mid (Autodesk Fusion 360 design; units mm, degrees)
Autodesk Fusion 360 part; units mm, degrees
note: some values were not read from the file. Set by a fixed rule: which sketch regions a step uses.
sketch "Sketch1" plane through (0, 0, 0) normal (0, 1, 0) x (1, 0, 0)
  line L0 (0, 0) -> (-60, 0)
  line L1 (-60, 0) -> (-60, -40)
  line L2 (-60, -40) -> (0, -40)
  line L3 (0, -40) -> (0, 0)
  spline S0 degree 2 poles (-31.401, -19.5282) (-31.401, -20.0578) (-31.6754, -20.3466) knots 0 0 0 1 1 1
  spline S1 degree 2 poles (-31.6754, -20.3466) (-31.9498, -20.6355) (-32.4457, -20.6355) knots 0 0 0 1 1 1
  spline S2 degree 2 poles (-32.4457, -20.6355) (-32.903, -20.6355) (-33.1534, -20.3563) knots 0 0 0 1 1 1
  spline S3 degree 2 poles (-33.1534, -20.3563) (-33.4037, -20.077) (-33.4037, -19.5667) knots 0 0 0 1 1 1
  line L4 (-33.4037, -19.5667) -> (-33.6011, -20.5296)
  spline S4 degree 2 poles (-33.6011, -20.5296) (-33.3652, -21.0254) (-32.9776, -21.2975) knots 0 0 0 1 1 1
  spline S5 degree 2 poles (-32.9776, -21.2975) (-32.5901, -21.5695) (-32.1231, -21.5695) knots 0 0 0 1 1 1
  spline S6 degree 2 poles (-32.1231, -21.5695) (-31.5839, -21.5695) (-31.2012, -21.3312) knots 0 0 0 1 1 1
  spline S7 degree 2 poles (-31.2012, -21.3312) (-30.8184, -21.0928) (-30.6186, -20.6355) knots 0 0 0 1 1 1
  spline S8 degree 2 poles (-30.6186, -20.6355) (-30.4188, -20.1781) (-30.4188, -19.533) knots 0 0 0 1 1 1
  line L5 (-30.4188, -19.533) -> (-30.4188, -16.5)
  line L6 (-30.4188, -16.5) -> (-31.401, -16.5)
  line L7 (-31.401, -16.5) -> (-31.401, -19.5282)
  line L8 (-37.3707, -21.4972) -> (-36.3886, -21.4972)
  line L9 (-36.3886, -21.4972) -> (-36.3886, -16.5)
  line L10 (-36.3886, -16.5) -> (-37.3707, -16.5)
  line L11 (-37.3707, -16.5) -> (-37.3707, -21.4972)
  spline S9 degree 2 poles (-34.3858, -19.5282) (-34.3858, -20.0578) (-34.6458, -20.3466) knots 0 0 0 1 1 1
  spline S10 degree 2 poles (-34.6458, -20.3466) (-34.9058, -20.6355) (-35.3824, -20.6355) knots 0 0 0 1 1 1
  spline S11 degree 2 poles (-35.3824, -20.6355) (-35.8638, -20.6355) (-36.1262, -20.3803) knots 0 0 0 1 1 1
  spline S12 degree 2 poles (-36.1262, -20.3803) (-36.3886, -20.1252) (-36.3886, -19.663) knots 0 0 0 1 1 1
  line L12 (-36.3886, -19.663) -> (-36.4897, -20.6259)
  spline S13 degree 2 poles (-36.4897, -20.6259) (-36.2586, -21.0784) (-35.8855, -21.3239) knots 0 0 0 1 1 1
  spline S14 degree 2 poles (-35.8855, -21.3239) (-35.5124, -21.5695) (-35.0598, -21.5695) knots 0 0 0 1 1 1
  spline S15 degree 2 poles (-35.0598, -21.5695) (-34.5351, -21.5695) (-34.1644, -21.3312) knots 0 0 0 1 1 1
  spline S16 degree 2 poles (-34.1644, -21.3312) (-33.7937, -21.0928) (-33.5987, -20.6355) knots 0 0 0 1 1 1
  spline S17 degree 2 poles (-33.5987, -20.6355) (-33.4037, -20.1781) (-33.4037, -19.533) knots 0 0 0 1 1 1
  line L13 (-33.4037, -19.533) -> (-33.4037, -16.5)
  line L14 (-33.4037, -16.5) -> (-34.3858, -16.5)
  line L15 (-34.3858, -16.5) -> (-34.3858, -19.5282)
  line L16 (-28.9264, -23.5) -> (-27.9443, -23.5)
  line L17 (-27.9443, -23.5) -> (-27.9443, -22.5179)
  line L18 (-27.9443, -22.5179) -> (-28.9264, -22.5179)
  line L19 (-28.9264, -22.5179) -> (-28.9264, -23.5)
  line L20 (-28.9264, -21.4972) -> (-27.9443, -21.4972)
  line L21 (-27.9443, -21.4972) -> (-27.9443, -16.5)
  line L22 (-27.9443, -16.5) -> (-28.9264, -16.5)
  line L23 (-28.9264, -16.5) -> (-28.9264, -21.4972)
  line L24 (-23.6114, -23.5) -> (-22.6293, -23.5)
  line L25 (-22.6293, -23.5) -> (-22.6293, -16.5)
  line L26 (-22.6293, -16.5) -> (-23.6114, -16.5)
  line L27 (-23.6114, -16.5) -> (-23.6114, -23.5)
  spline S18 degree 2 poles (-24.868, -16.4133) (-25.4168, -16.4133) (-25.8043, -16.6516) knots 0 0 0 1 1 1
  spline S19 degree 2 poles (-25.8043, -16.6516) (-26.1919, -16.89) (-26.3941, -17.3473) knots 0 0 0 1 1 1
  spline S20 degree 2 poles (-26.3941, -17.3473) (-26.5963, -17.8047) (-26.5963, -18.445) knots 0 0 0 1 1 1
  line L28 (-26.5963, -18.445) -> (-26.5963, -19.5475)
  spline S21 degree 2 poles (-26.5963, -19.5475) (-26.5963, -20.1926) (-26.3989, -20.6499) knots 0 0 0 1 1 1
  spline S22 degree 2 poles (-26.3989, -20.6499) (-26.2015, -21.1073) (-25.8236, -21.3456) knots 0 0 0 1 1 1
  spline S23 degree 2 poles (-25.8236, -21.3456) (-25.4457, -21.5839) (-24.9161, -21.5839) knots 0 0 0 1 1 1
  spline S24 degree 2 poles (-24.9161, -21.5839) (-24.4732, -21.5839) (-24.1049, -21.3528) knots 0 0 0 1 1 1
  spline S25 degree 2 poles (-24.1049, -21.3528) (-23.7366, -21.1217) (-23.5103, -20.7029) knots 0 0 0 1 1 1
  line L29 (-23.5103, -20.7029) -> (-23.6114, -19.6823)
  spline S26 degree 2 poles (-23.6114, -19.6823) (-23.6114, -20) (-23.727, -20.2263) knots 0 0 0 1 1 1
  spline S27 degree 2 poles (-23.727, -20.2263) (-23.8425, -20.4525) (-24.0616, -20.5705) knots 0 0 0 1 1 1
  spline S28 degree 2 poles (-24.0616, -20.5705) (-24.2806, -20.6884) (-24.5935, -20.6884) knots 0 0 0 1 1 1
  spline S29 degree 2 poles (-24.5935, -20.6884) (-25.0798, -20.6884) (-25.347, -20.3851) knots 0 0 0 1 1 1
  spline S30 degree 2 poles (-25.347, -20.3851) (-25.6142, -20.0818) (-25.6142, -19.533) knots 0 0 0 1 1 1
  line L30 (-25.6142, -19.533) -> (-25.6142, -18.445)
  spline S31 degree 2 poles (-25.6142, -18.445) (-25.6142, -17.901) (-25.347, -17.6049) knots 0 0 0 1 1 1
  spline S32 degree 2 poles (-25.347, -17.6049) (-25.0798, -17.3088) (-24.5935, -17.3088) knots 0 0 0 1 1 1
  spline S33 degree 2 poles (-24.5935, -17.3088) (-24.2806, -17.3088) (-24.0616, -17.4316) knots 0 0 0 1 1 1
  spline S34 degree 2 poles (-24.0616, -17.4316) (-23.8425, -17.5543) (-23.727, -17.7854) knots 0 0 0 1 1 1
  spline S35 degree 2 poles (-23.727, -17.7854) (-23.6114, -18.0165) (-23.6114, -18.3391) knots 0 0 0 1 1 1
  line L31 (-23.6114, -18.3391) -> (-23.544, -17.2847)
  spline S36 degree 2 poles (-23.544, -17.2847) (-23.6933, -16.914) (-24.0327, -16.6637) knots 0 0 0 1 1 1
  spline S37 degree 2 poles (-24.0327, -16.6637) (-24.3721, -16.4133) (-24.868, -16.4133) knots 0 0 0 1 1 1
  line L32 (0, 5) -> (-60, 5)
  line L33 (-60, 5) -> (-60, 33)
  line L34 (-60, 33) -> (0, 33)
  line L35 (0, 33) -> (0, 5)
  spline S38 degree 2 poles (-47.8102, 16.7607) (-48.641, 16.7607) (-49.271, 16.392) knots 0 0 0 1 1 1
  spline S39 degree 2 poles (-49.271, 16.392) (-49.901, 16.0234) (-50.2476, 15.3466) knots 0 0 0 1 1 1
  spline S40 degree 2 poles (-50.2476, 15.3466) (-50.5942, 14.6699) (-50.5942, 13.7785) knots 0 0 0 1 1 1
  line L36 (-50.5942, 13.7785) -> (-50.5942, 11.5832)
  spline S41 degree 2 poles (-50.5942, 11.5832) (-50.5942, 10.6919) (-50.2476, 10.0151) knots 0 0 0 1 1 1
  spline S42 degree 2 poles (-50.2476, 10.0151) (-49.901, 9.3384) (-49.271, 8.967) knots 0 0 0 1 1 1
  spline S43 degree 2 poles (-49.271, 8.967) (-48.641, 8.5956) (-47.8102, 8.5956) knots 0 0 0 1 1 1
  spline S44 degree 2 poles (-47.8102, 8.5956) (-47.1224, 8.5956) (-46.5447, 8.89) knots 0 0 0 1 1 1
  spline S45 degree 2 poles (-46.5447, 8.89) (-45.967, 9.1843) (-45.5791, 9.7235) knots 0 0 0 1 1 1
  spline S46 degree 2 poles (-45.5791, 9.7235) (-45.1912, 10.2627) (-45.0536, 10.9725) knots 0 0 0 1 1 1
  line L37 (-45.0536, 10.9725) -> (-46.2036, 10.9725)
  spline S47 degree 2 poles (-46.2036, 10.9725) (-46.3081, 10.5983) (-46.553, 10.304) knots 0 0 0 1 1 1
  spline S48 degree 2 poles (-46.553, 10.304) (-46.7978, 10.0096) (-47.1279, 9.8501) knots 0 0 0 1 1 1
  spline S49 degree 2 poles (-47.1279, 9.8501) (-47.458, 9.6905) (-47.8102, 9.6905) knots 0 0 0 1 1 1
  spline S50 degree 2 poles (-47.8102, 9.6905) (-48.2999, 9.6905) (-48.6685, 9.9271) knots 0 0 0 1 1 1
  spline S51 degree 2 poles (-48.6685, 9.9271) (-49.0371, 10.1637) (-49.2407, 10.5901) knots 0 0 0 1 1 1
  spline S52 degree 2 poles (-49.2407, 10.5901) (-49.4443, 11.0165) (-49.4443, 11.5832) knots 0 0 0 1 1 1
  line L38 (-49.4443, 11.5832) -> (-49.4443, 13.7785)
  spline S53 degree 2 poles (-49.4443, 13.7785) (-49.4443, 14.3398) (-49.2407, 14.7689) knots 0 0 0 1 1 1
  spline S54 degree 2 poles (-49.2407, 14.7689) (-49.0371, 15.1981) (-48.6685, 15.4319) knots 0 0 0 1 1 1
  spline S55 degree 2 poles (-48.6685, 15.4319) (-48.2999, 15.6657) (-47.8102, 15.6657) knots 0 0 0 1 1 1
  spline S56 degree 2 poles (-47.8102, 15.6657) (-47.4525, 15.6657) (-47.1252, 15.5172) knots 0 0 0 1 1 1
  spline S57 degree 2 poles (-47.1252, 15.5172) (-46.7978, 15.3686) (-46.553, 15.077) knots 0 0 0 1 1 1
  spline S58 degree 2 poles (-46.553, 15.077) (-46.3081, 14.7854) (-46.2036, 14.3838) knots 0 0 0 1 1 1
  line L39 (-46.2036, 14.3838) -> (-45.0536, 14.3838)
  spline S59 degree 2 poles (-45.0536, 14.3838) (-45.1912, 15.0935) (-45.5818, 15.6327) knots 0 0 0 1 1 1
  spline S60 degree 2 poles (-45.5818, 15.6327) (-45.9725, 16.1719) (-46.5502, 16.4663) knots 0 0 0 1 1 1
  spline S61 degree 2 poles (-46.5502, 16.4663) (-47.1279, 16.7607) (-47.8102, 16.7607) knots 0 0 0 1 1 1
  spline S62 degree 2 poles (-41.2297, 16.7607) (-42.022, 16.7607) (-42.5832, 16.4635) knots 0 0 0 1 1 1
  spline S63 degree 2 poles (-42.5832, 16.4635) (-43.1444, 16.1664) (-43.4388, 15.5915) knots 0 0 0 1 1 1
  spline S64 degree 2 poles (-43.4388, 15.5915) (-43.7332, 15.0165) (-43.7332, 14.2022) knots 0 0 0 1 1 1
  line L40 (-43.7332, 14.2022) -> (-43.7332, 13.5585)
  spline S65 degree 2 poles (-43.7332, 13.5585) (-43.7332, 12.7111) (-43.4498, 12.1114) knots 0 0 0 1 1 1
  spline S66 degree 2 poles (-43.4498, 12.1114) (-43.1664, 11.5117) (-42.6272, 11.1981) knots 0 0 0 1 1 1
  spline S67 degree 2 poles (-42.6272, 11.1981) (-42.088, 10.8845) (-41.3287, 10.8845) knots 0 0 0 1 1 1
  spline S68 degree 2 poles (-41.3287, 10.8845) (-40.6135, 10.8845) (-40.1073, 11.2421) knots 0 0 0 1 1 1
  spline S69 degree 2 poles (-40.1073, 11.2421) (-39.6011, 11.5997) (-39.3343, 12.2765) knots 0 0 0 1 1 1
  spline S70 degree 2 poles (-39.3343, 12.2765) (-39.0674, 12.9532) (-39.0674, 13.8996) knots 0 0 0 1 1 1
  line L41 (-39.0674, 13.8996) -> (-39.0674, 14.2737)
  line L42 (-39.0674, 14.2737) -> (-42.9188, 14.2737)
  line L43 (-42.9188, 14.2737) -> (-42.9188, 13.3714)
  line L44 (-42.9188, 13.3714) -> (-40.1348, 13.3714)
  spline S71 degree 2 poles (-40.1348, 13.3714) (-40.1843, 12.6726) (-40.4952, 12.2847) knots 0 0 0 1 1 1
  spline S72 degree 2 poles (-40.4952, 12.2847) (-40.8061, 11.8968) (-41.3287, 11.8968) knots 0 0 0 1 1 1
  spline S73 degree 2 poles (-41.3287, 11.8968) (-41.967, 11.8968) (-42.3164, 12.315) knots 0 0 0 1 1 1
  spline S74 degree 2 poles (-42.3164, 12.315) (-42.6658, 12.7332) (-42.6658, 13.4979) knots 0 0 0 1 1 1
  line L45 (-42.6658, 13.4979) -> (-42.6658, 14.2242)
  spline S75 degree 2 poles (-42.6658, 14.2242) (-42.6658, 14.934) (-42.2916, 15.3136) knots 0 0 0 1 1 1
  spline S76 degree 2 poles (-42.2916, 15.3136) (-41.9175, 15.6933) (-41.2297, 15.6933) knots 0 0 0 1 1 1
  spline S77 degree 2 poles (-41.2297, 15.6933) (-40.8886, 15.6933) (-40.553, 15.5557) knots 0 0 0 1 1 1
  spline S78 degree 2 poles (-40.553, 15.5557) (-40.2173, 15.4182) (-39.9532, 15.1706) knots 0 0 0 1 1 1
  line L46 (-39.9532, 15.1706) -> (-39.216, 15.9078)
  spline S79 degree 2 poles (-39.216, 15.9078) (-39.6396, 16.315) (-40.1678, 16.5378) knots 0 0 0 1 1 1
  spline S80 degree 2 poles (-40.1678, 16.5378) (-40.696, 16.7607) (-41.2297, 16.7607) knots 0 0 0 1 1 1
  line L47 (-37.5268, 10.967) -> (-36.4044, 10.967)
  line L48 (-36.4044, 10.967) -> (-36.4044, 16.6781)
  line L49 (-36.4044, 16.6781) -> (-37.5268, 16.6781)
  line L50 (-37.5268, 16.6781) -> (-37.5268, 10.967)
  spline S81 degree 2 poles (-34.3851, 12.3205) (-34.5337, 12.1389) (-34.7593, 12.0454) knots 0 0 0 1 1 1
  spline S82 degree 2 poles (-34.7593, 12.0454) (-34.9849, 11.9519) (-35.282, 11.9519) knots 0 0 0 1 1 1
  spline S83 degree 2 poles (-35.282, 11.9519) (-35.8157, 11.9519) (-36.11, 12.2462) knots 0 0 0 1 1 1
  spline S84 degree 2 poles (-36.11, 12.2462) (-36.4044, 12.5406) (-36.4044, 13.0633) knots 0 0 0 1 1 1
  line L51 (-36.4044, 13.0633) -> (-36.5199, 11.9629)
  spline S85 degree 2 poles (-36.5199, 11.9629) (-36.2558, 11.4512) (-35.8377, 11.1678) knots 0 0 0 1 1 1
  spline S86 degree 2 poles (-35.8377, 11.1678) (-35.4195, 10.8845) (-34.9133, 10.8845) knots 0 0 0 1 1 1
  spline S87 degree 2 poles (-34.9133, 10.8845) (-34.5227, 10.8845) (-34.2063, 10.9972) knots 0 0 0 1 1 1
  spline S88 degree 2 poles (-34.2063, 10.9972) (-33.89, 11.11) (-33.6534, 11.3301) knots 0 0 0 1 1 1
  line L52 (-33.6534, 11.3301) -> (-34.3851, 12.3205)
  spline S89 degree 2 poles (-31.2325, 16.7056) (-31.9257, 16.7056) (-32.2476, 16.3232) knots 0 0 0 1 1 1
  spline S90 degree 2 poles (-32.2476, 16.3232) (-32.5695, 15.9409) (-32.5695, 15.1926) knots 0 0 0 1 1 1
  line L53 (-32.5695, 15.1926) -> (-32.5695, 9.3054)
  line L54 (-32.5695, 9.3054) -> (-31.447, 9.3054)
  line L55 (-31.447, 9.3054) -> (-31.447, 15.2036)
  spline S91 degree 2 poles (-31.447, 15.2036) (-31.447, 15.4127) (-31.3645, 15.5254) knots 0 0 0 1 1 1
  spline S92 degree 2 poles (-31.3645, 15.5254) (-31.282, 15.6382) (-31.1224, 15.6382) knots 0 0 0 1 1 1
  line L56 (-31.1224, 15.6382) -> (-30.5832, 15.6382)
  line L57 (-30.5832, 15.6382) -> (-30.5832, 16.7056)
  line L58 (-30.5832, 16.7056) -> (-31.2325, 16.7056)
  line L59 (-33.1582, 10.967) -> (-30.5832, 10.967)
  line L60 (-30.5832, 10.967) -> (-30.5832, 11.9794)
  line L61 (-30.5832, 11.9794) -> (-33.1582, 11.9794)
  line L62 (-33.1582, 11.9794) -> (-33.1582, 10.967)
  line L63 (-29.0426, 8.6781) -> (-27.9202, 8.6781)
  line L64 (-27.9202, 8.6781) -> (-27.9202, 9.8006)
  line L65 (-27.9202, 9.8006) -> (-29.0426, 9.8006)
  line L66 (-29.0426, 9.8006) -> (-29.0426, 8.6781)
  line L67 (-29.0426, 10.967) -> (-27.9202, 10.967)
  line L68 (-27.9202, 10.967) -> (-27.9202, 16.6781)
  line L69 (-27.9202, 16.6781) -> (-29.0426, 16.6781)
  line L70 (-29.0426, 16.6781) -> (-29.0426, 10.967)
  spline S93 degree 2 poles (-26.0495, 10.1912) (-26.0495, 9.4319) (-25.7001, 9.055) knots 0 0 0 1 1 1
  spline S94 degree 2 poles (-25.7001, 9.055) (-25.3508, 8.6781) (-24.6245, 8.6781) knots 0 0 0 1 1 1
  line L71 (-24.6245, 8.6781) -> (-23.7992, 8.6781)
  line L72 (-23.7992, 8.6781) -> (-23.7992, 9.7455)
  line L73 (-23.7992, 9.7455) -> (-24.6025, 9.7455)
  spline S95 degree 2 poles (-24.6025, 9.7455) (-24.762, 9.7455) (-24.8446, 9.8666) knots 0 0 0 1 1 1
  spline S96 degree 2 poles (-24.8446, 9.8666) (-24.9271, 9.9876) (-24.9271, 10.1802) knots 0 0 0 1 1 1
  line L74 (-24.9271, 10.1802) -> (-24.9271, 16.6781)
  line L75 (-24.9271, 16.6781) -> (-26.0495, 16.6781)
  line L76 (-26.0495, 16.6781) -> (-26.0495, 10.1912)
  line L77 (-26.6547, 10.967) -> (-23.7992, 10.967)
  line L78 (-23.7992, 10.967) -> (-23.7992, 11.9243)
  line L79 (-23.7992, 11.9243) -> (-26.6547, 11.9243)
  line L80 (-26.6547, 11.9243) -> (-26.6547, 10.967)
  line L81 (-22.6437, 8.6781) -> (-21.5213, 8.6781)
  line L82 (-21.5213, 8.6781) -> (-21.5213, 9.8006)
  line L83 (-21.5213, 9.8006) -> (-22.6437, 9.8006)
  line L84 (-22.6437, 9.8006) -> (-22.6437, 8.6781)
  line L85 (-22.6437, 10.967) -> (-21.5213, 10.967)
  line L86 (-21.5213, 10.967) -> (-21.5213, 16.6781)
  line L87 (-21.5213, 16.6781) -> (-22.6437, 16.6781)
  line L88 (-22.6437, 16.6781) -> (-22.6437, 10.967)
  spline S97 degree 2 poles (-17.4773, 16.7607) (-18.2696, 16.7607) (-18.8308, 16.4635) knots 0 0 0 1 1 1
  spline S98 degree 2 poles (-18.8308, 16.4635) (-19.392, 16.1664) (-19.6864, 15.5915) knots 0 0 0 1 1 1
  spline S99 degree 2 poles (-19.6864, 15.5915) (-19.9807, 15.0165) (-19.9807, 14.2022) knots 0 0 0 1 1 1
  line L89 (-19.9807, 14.2022) -> (-19.9807, 13.5585)
  spline S100 degree 2 poles (-19.9807, 13.5585) (-19.9807, 12.7111) (-19.6974, 12.1114) knots 0 0 0 1 1 1
  spline S101 degree 2 poles (-19.6974, 12.1114) (-19.414, 11.5117) (-18.8748, 11.1981) knots 0 0 0 1 1 1
  spline S102 degree 2 poles (-18.8748, 11.1981) (-18.3356, 10.8845) (-17.5763, 10.8845) knots 0 0 0 1 1 1
  spline S103 degree 2 poles (-17.5763, 10.8845) (-16.8611, 10.8845) (-16.3549, 11.2421) knots 0 0 0 1 1 1
  spline S104 degree 2 poles (-16.3549, 11.2421) (-15.8487, 11.5997) (-15.5818, 12.2765) knots 0 0 0 1 1 1
  spline S105 degree 2 poles (-15.5818, 12.2765) (-15.315, 12.9532) (-15.315, 13.8996) knots 0 0 0 1 1 1
  line L90 (-15.315, 13.8996) -> (-15.315, 14.2737)
  line L91 (-15.315, 14.2737) -> (-19.1664, 14.2737)
  line L92 (-19.1664, 14.2737) -> (-19.1664, 13.3714)
  line L93 (-19.1664, 13.3714) -> (-16.3824, 13.3714)
  spline S106 degree 2 poles (-16.3824, 13.3714) (-16.4319, 12.6726) (-16.7428, 12.2847) knots 0 0 0 1 1 1
  spline S107 degree 2 poles (-16.7428, 12.2847) (-17.0536, 11.8968) (-17.5763, 11.8968) knots 0 0 0 1 1 1
  spline S108 degree 2 poles (-17.5763, 11.8968) (-18.2146, 11.8968) (-18.564, 12.315) knots 0 0 0 1 1 1
  spline S109 degree 2 poles (-18.564, 12.315) (-18.9133, 12.7332) (-18.9133, 13.4979) knots 0 0 0 1 1 1
  line L94 (-18.9133, 13.4979) -> (-18.9133, 14.2242)
  spline S110 degree 2 poles (-18.9133, 14.2242) (-18.9133, 14.934) (-18.5392, 15.3136) knots 0 0 0 1 1 1
  spline S111 degree 2 poles (-18.5392, 15.3136) (-18.1651, 15.6933) (-17.4773, 15.6933) knots 0 0 0 1 1 1
  spline S112 degree 2 poles (-17.4773, 15.6933) (-17.1362, 15.6933) (-16.8005, 15.5557) knots 0 0 0 1 1 1
  spline S113 degree 2 poles (-16.8005, 15.5557) (-16.4649, 15.4182) (-16.2008, 15.1706) knots 0 0 0 1 1 1
  line L95 (-16.2008, 15.1706) -> (-15.4636, 15.9078)
  spline S114 degree 2 poles (-15.4636, 15.9078) (-15.8872, 16.315) (-16.4154, 16.5378) knots 0 0 0 1 1 1
  spline S115 degree 2 poles (-16.4154, 16.5378) (-16.9436, 16.7607) (-17.4773, 16.7607) knots 0 0 0 1 1 1
  line L96 (-10.5282, 8.6781) -> (-9.4058, 8.6781)
  line L97 (-9.4058, 8.6781) -> (-9.4058, 16.6781)
  line L98 (-9.4058, 16.6781) -> (-10.5282, 16.6781)
  line L99 (-10.5282, 16.6781) -> (-10.5282, 8.6781)
  spline S116 degree 2 poles (-11.9642, 16.7772) (-12.5915, 16.7772) (-13.0344, 16.5048) knots 0 0 0 1 1 1
  spline S117 degree 2 poles (-13.0344, 16.5048) (-13.4773, 16.2325) (-13.7084, 15.7098) knots 0 0 0 1 1 1
  spline S118 degree 2 poles (-13.7084, 15.7098) (-13.9395, 15.1871) (-13.9395, 14.4553) knots 0 0 0 1 1 1
  line L100 (-13.9395, 14.4553) -> (-13.9395, 13.1953)
  spline S119 degree 2 poles (-13.9395, 13.1953) (-13.9395, 12.458) (-13.7139, 11.9354) knots 0 0 0 1 1 1
  spline S120 degree 2 poles (-13.7139, 11.9354) (-13.4883, 11.4127) (-13.0564, 11.1403) knots 0 0 0 1 1 1
  spline S121 degree 2 poles (-13.0564, 11.1403) (-12.6245, 10.868) (-12.0193, 10.868) knots 0 0 0 1 1 1
  spline S122 degree 2 poles (-12.0193, 10.868) (-11.5131, 10.868) (-11.0922, 11.132) knots 0 0 0 1 1 1
  spline S123 degree 2 poles (-11.0922, 11.132) (-10.6713, 11.3961) (-10.4127, 11.8748) knots 0 0 0 1 1 1
  line L101 (-10.4127, 11.8748) -> (-10.5282, 13.0413)
  spline S124 degree 2 poles (-10.5282, 13.0413) (-10.5282, 12.6781) (-10.6602, 12.4195) knots 0 0 0 1 1 1
  spline S125 degree 2 poles (-10.6602, 12.4195) (-10.7923, 12.1609) (-11.0426, 12.0261) knots 0 0 0 1 1 1
  spline S126 degree 2 poles (-11.0426, 12.0261) (-11.293, 11.8913) (-11.6506, 11.8913) knots 0 0 0 1 1 1
  spline S127 degree 2 poles (-11.6506, 11.8913) (-12.2063, 11.8913) (-12.5117, 12.238) knots 0 0 0 1 1 1
  spline S128 degree 2 poles (-12.5117, 12.238) (-12.8171, 12.5846) (-12.8171, 13.2118) knots 0 0 0 1 1 1
  line L102 (-12.8171, 13.2118) -> (-12.8171, 14.4553)
  spline S129 degree 2 poles (-12.8171, 14.4553) (-12.8171, 15.077) (-12.5117, 15.4154) knots 0 0 0 1 1 1
  spline S130 degree 2 poles (-12.5117, 15.4154) (-12.2063, 15.7538) (-11.6506, 15.7538) knots 0 0 0 1 1 1
  spline S131 degree 2 poles (-11.6506, 15.7538) (-11.293, 15.7538) (-11.0426, 15.6135) knots 0 0 0 1 1 1
  spline S132 degree 2 poles (-11.0426, 15.6135) (-10.7923, 15.4732) (-10.6602, 15.2091) knots 0 0 0 1 1 1
  spline S133 degree 2 poles (-10.6602, 15.2091) (-10.5282, 14.945) (-10.5282, 14.5763) knots 0 0 0 1 1 1
  line L103 (-10.5282, 14.5763) -> (-10.4512, 15.7813)
  spline S134 degree 2 poles (-10.4512, 15.7813) (-10.6217, 16.205) (-11.0096, 16.4911) knots 0 0 0 1 1 1
  spline S135 degree 2 poles (-11.0096, 16.4911) (-11.3975, 16.7772) (-11.9642, 16.7772) knots 0 0 0 1 1 1
  line L104 (-55.2407, 29.1623) -> (-53.0729, 29.1623)
  spline S136 degree 2 poles (-53.0729, 29.1623) (-52.2201, 29.1623) (-51.8294, 28.8377) knots 0 0 0 1 1 1
  spline S137 degree 2 poles (-51.8294, 28.8377) (-51.4388, 28.5131) (-51.4388, 27.9243) knots 0 0 0 1 1 1
  line L105 (-51.4388, 27.9243) -> (-51.4388, 27.9078)
  spline S138 degree 2 poles (-51.4388, 27.9078) (-51.4388, 27.5007) (-51.5791, 27.2091) knots 0 0 0 1 1 1
  spline S139 degree 2 poles (-51.5791, 27.2091) (-51.7194, 26.9175) (-52.022, 26.7607) knots 0 0 0 1 1 1
  spline S140 degree 2 poles (-52.022, 26.7607) (-52.3246, 26.6039) (-52.7978, 26.6039) knots 0 0 0 1 1 1
  line L106 (-52.7978, 26.6039) -> (-55.2407, 26.6039)
  line L107 (-55.2407, 26.6039) -> (-55.2407, 25.5915)
  line L108 (-55.2407, 25.5915) -> (-52.7978, 25.5915)
  spline S141 degree 2 poles (-52.7978, 25.5915) (-52.1761, 25.5915) (-51.8597, 25.2999) knots 0 0 0 1 1 1
  spline S142 degree 2 poles (-51.8597, 25.2999) (-51.5433, 25.0083) (-51.5433, 24.436) knots 0 0 0 1 1 1
  spline S143 degree 2 poles (-51.5433, 24.436) (-51.5433, 23.8363) (-51.8955, 23.5392) knots 0 0 0 1 1 1
  spline S144 degree 2 poles (-51.8955, 23.5392) (-52.2476, 23.2421) (-52.9519, 23.2421) knots 0 0 0 1 1 1
  line L109 (-52.9519, 23.2421) -> (-55.2407, 23.2421)
  line L110 (-55.2407, 23.2421) -> (-55.2407, 22.2022)
  line L111 (-55.2407, 22.2022) -> (-52.7483, 22.2022)
  spline S145 degree 2 poles (-52.7483, 22.2022) (-51.9725, 22.2022) (-51.4498, 22.4663) knots 0 0 0 1 1 1
  spline S146 degree 2 poles (-51.4498, 22.4663) (-50.9271, 22.7304) (-50.6685, 23.2146) knots 0 0 0 1 1 1
  spline S147 degree 2 poles (-50.6685, 23.2146) (-50.4099, 23.6988) (-50.4099, 24.37) knots 0 0 0 1 1 1
  spline S148 degree 2 poles (-50.4099, 24.37) (-50.4099, 24.7827) (-50.5695, 25.1431) knots 0 0 0 1 1 1
  spline S149 degree 2 poles (-50.5695, 25.1431) (-50.729, 25.5034) (-51.0564, 25.7593) knots 0 0 0 1 1 1
  spline S150 degree 2 poles (-51.0564, 25.7593) (-51.3838, 26.0151) (-51.868, 26.1032) knots 0 0 0 1 1 1
  spline S151 degree 2 poles (-51.868, 26.1032) (-51.3838, 26.1747) (-51.0316, 26.447) knots 0 0 0 1 1 1
  spline S152 degree 2 poles (-51.0316, 26.447) (-50.6795, 26.7194) (-50.4924, 27.1265) knots 0 0 0 1 1 1
  spline S153 degree 2 poles (-50.4924, 27.1265) (-50.3054, 27.5337) (-50.3054, 28.0069) knots 0 0 0 1 1 1
  line L112 (-50.3054, 28.0069) -> (-50.3054, 28.0234)
  spline S154 degree 2 poles (-50.3054, 28.0234) (-50.3054, 28.6726) (-50.5915, 29.1678) knots 0 0 0 1 1 1
  spline S155 degree 2 poles (-50.5915, 29.1678) (-50.8776, 29.663) (-51.4113, 29.9326) knots 0 0 0 1 1 1
  spline S156 degree 2 poles (-51.4113, 29.9326) (-51.945, 30.2022) (-52.6547, 30.2022) knots 0 0 0 1 1 1
  line L113 (-52.6547, 30.2022) -> (-55.2407, 30.2022)
  line L114 (-55.2407, 30.2022) -> (-55.2407, 29.1623)
  line L115 (-55.901, 22.2022) -> (-54.784, 22.2022)
  line L116 (-54.784, 22.2022) -> (-54.784, 30.2022)
  line L117 (-54.784, 30.2022) -> (-55.901, 30.2022)
  line L118 (-55.901, 30.2022) -> (-55.901, 22.2022)
  spline S157 degree 2 poles (-45.5131, 26.5818) (-45.5131, 26.0206) (-45.8129, 25.7098) knots 0 0 0 1 1 1
  spline S158 degree 2 poles (-45.8129, 25.7098) (-46.1128, 25.3989) (-46.663, 25.3989) knots 0 0 0 1 1 1
  spline S159 degree 2 poles (-46.663, 25.3989) (-47.0041, 25.3989) (-47.3315, 25.5034) knots 0 0 0 1 1 1
  spline S160 degree 2 poles (-47.3315, 25.5034) (-47.6589, 25.608) (-47.912, 25.795) knots 0 0 0 1 1 1
  line L119 (-47.912, 25.795) -> (-48.7318, 25.2338)
  spline S161 degree 2 poles (-48.7318, 25.2338) (-48.4072, 24.8432) (-47.8762, 24.6259) knots 0 0 0 1 1 1
  spline S162 degree 2 poles (-47.8762, 24.6259) (-47.3453, 24.4085) (-46.696, 24.4085) knots 0 0 0 1 1 1
  spline S163 degree 2 poles (-46.696, 24.4085) (-45.9862, 24.4085) (-45.4801, 24.6589) knots 0 0 0 1 1 1
  spline S164 degree 2 poles (-45.4801, 24.6589) (-44.9739, 24.9092) (-44.7098, 25.3851) knots 0 0 0 1 1 1
  spline S165 degree 2 poles (-44.7098, 25.3851) (-44.4457, 25.8611) (-44.4457, 26.5323) knots 0 0 0 1 1 1
  line L120 (-44.4457, 26.5323) -> (-44.4457, 30.2022)
  line L121 (-44.4457, 30.2022) -> (-45.5131, 30.2022)
  line L122 (-45.5131, 30.2022) -> (-45.5131, 26.5818)
  spline S166 degree 2 poles (-46.9106, 30.2847) (-47.967, 30.2847) (-48.4897, 29.8473) knots 0 0 0 1 1 1
  spline S167 degree 2 poles (-48.4897, 29.8473) (-49.0124, 29.4099) (-49.0124, 28.5186) knots 0 0 0 1 1 1
  spline S168 degree 2 poles (-49.0124, 28.5186) (-49.0124, 27.6713) (-48.5337, 27.2476) knots 0 0 0 1 1 1
  spline S169 degree 2 poles (-48.5337, 27.2476) (-48.055, 26.8239) (-47.0867, 26.8239) knots 0 0 0 1 1 1
  line L123 (-47.0867, 26.8239) -> (-45.4636, 26.8239)
  line L124 (-45.4636, 26.8239) -> (-45.3865, 27.7263)
  line L125 (-45.3865, 27.7263) -> (-47.0812, 27.7263)
  spline S170 degree 2 poles (-47.0812, 27.7263) (-47.5213, 27.7263) (-47.7387, 27.9216) knots 0 0 0 1 1 1
  spline S171 degree 2 poles (-47.7387, 27.9216) (-47.956, 28.1169) (-47.956, 28.5186) knots 0 0 0 1 1 1
  spline S172 degree 2 poles (-47.956, 28.5186) (-47.956, 28.9532) (-47.6671, 29.1623) knots 0 0 0 1 1 1
  spline S173 degree 2 poles (-47.6671, 29.1623) (-47.3783, 29.3714) (-46.7895, 29.3714) knots 0 0 0 1 1 1
  spline S174 degree 2 poles (-46.7895, 29.3714) (-46.1458, 29.3714) (-45.8294, 29.2338) knots 0 0 0 1 1 1
  spline S175 degree 2 poles (-45.8294, 29.2338) (-45.5131, 29.0963) (-45.5131, 28.8047) knots 0 0 0 1 1 1
  line L126 (-45.5131, 28.8047) -> (-45.3975, 29.608)
  spline S176 degree 2 poles (-45.3975, 29.608) (-45.5461, 29.8391) (-45.7634, 29.9876) knots 0 0 0 1 1 1
  spline S177 degree 2 poles (-45.7634, 29.9876) (-45.9807, 30.1362) (-46.2669, 30.2105) knots 0 0 0 1 1 1
  spline S178 degree 2 poles (-46.2669, 30.2105) (-46.553, 30.2847) (-46.9106, 30.2847) knots 0 0 0 1 1 1
  line L127 (-39.4938, 22.2022) -> (-38.3714, 22.2022)
  line L128 (-38.3714, 22.2022) -> (-38.3714, 30.2022)
  line L129 (-38.3714, 30.2022) -> (-39.4938, 30.2022)
  line L130 (-39.4938, 30.2022) -> (-39.4938, 22.2022)
  spline S179 degree 2 poles (-40.9299, 30.3012) (-41.5571, 30.3012) (-42, 30.0289) knots 0 0 0 1 1 1
  spline S180 degree 2 poles (-42, 30.0289) (-42.4429, 29.7565) (-42.674, 29.2338) knots 0 0 0 1 1 1
  spline S181 degree 2 poles (-42.674, 29.2338) (-42.9051, 28.7111) (-42.9051, 27.9794) knots 0 0 0 1 1 1
  line L131 (-42.9051, 27.9794) -> (-42.9051, 26.7194)
  spline S182 degree 2 poles (-42.9051, 26.7194) (-42.9051, 25.9821) (-42.6795, 25.4594) knots 0 0 0 1 1 1
  spline S183 degree 2 poles (-42.6795, 25.4594) (-42.4539, 24.9367) (-42.022, 24.6644) knots 0 0 0 1 1 1
  spline S184 degree 2 poles (-42.022, 24.6644) (-41.5901, 24.392) (-40.9849, 24.392) knots 0 0 0 1 1 1
  spline S185 degree 2 poles (-40.9849, 24.392) (-40.4787, 24.392) (-40.0578, 24.6561) knots 0 0 0 1 1 1
  spline S186 degree 2 poles (-40.0578, 24.6561) (-39.6369, 24.9202) (-39.3783, 25.3989) knots 0 0 0 1 1 1
  line L132 (-39.3783, 25.3989) -> (-39.4938, 26.5653)
  spline S187 degree 2 poles (-39.4938, 26.5653) (-39.4938, 26.2022) (-39.6259, 25.9436) knots 0 0 0 1 1 1
  spline S188 degree 2 poles (-39.6259, 25.9436) (-39.7579, 25.685) (-40.0083, 25.5502) knots 0 0 0 1 1 1
  spline S189 degree 2 poles (-40.0083, 25.5502) (-40.2586, 25.4154) (-40.6162, 25.4154) knots 0 0 0 1 1 1
  spline S190 degree 2 poles (-40.6162, 25.4154) (-41.1719, 25.4154) (-41.4773, 25.762) knots 0 0 0 1 1 1
  spline S191 degree 2 poles (-41.4773, 25.762) (-41.7827, 26.1087) (-41.7827, 26.7359) knots 0 0 0 1 1 1
  line L133 (-41.7827, 26.7359) -> (-41.7827, 27.9794)
  spline S192 degree 2 poles (-41.7827, 27.9794) (-41.7827, 28.6011) (-41.4773, 28.9395) knots 0 0 0 1 1 1
  spline S193 degree 2 poles (-41.4773, 28.9395) (-41.1719, 29.2779) (-40.6162, 29.2779) knots 0 0 0 1 1 1
  spline S194 degree 2 poles (-40.6162, 29.2779) (-40.2586, 29.2779) (-40.0083, 29.1376) knots 0 0 0 1 1 1
  spline S195 degree 2 poles (-40.0083, 29.1376) (-39.7579, 28.9972) (-39.6259, 28.7331) knots 0 0 0 1 1 1
  spline S196 degree 2 poles (-39.6259, 28.7331) (-39.4938, 28.469) (-39.4938, 28.1004) knots 0 0 0 1 1 1
  line L134 (-39.4938, 28.1004) -> (-39.4168, 29.3054)
  spline S197 degree 2 poles (-39.4168, 29.3054) (-39.5873, 29.729) (-39.9752, 30.0151) knots 0 0 0 1 1 1
  spline S198 degree 2 poles (-39.9752, 30.0151) (-40.3631, 30.3012) (-40.9299, 30.3012) knots 0 0 0 1 1 1
  line L135 (-32.3686, 22.8569) -> (-31.2462, 22.8569)
  line L136 (-31.2462, 22.8569) -> (-31.2462, 30.2022)
  line L137 (-31.2462, 30.2022) -> (-32.3686, 30.2022)
  line L138 (-32.3686, 30.2022) -> (-32.3686, 22.8569)
  line L139 (-34.63, 22.2022) -> (-28.9849, 22.2022)
  line L140 (-28.9849, 22.2022) -> (-28.9849, 23.2696)
  line L141 (-28.9849, 23.2696) -> (-34.63, 23.2696)
  line L142 (-34.63, 23.2696) -> (-34.63, 22.2022)
  line L143 (-28.2146, 22.2022) -> (-27.0922, 22.2022)
  line L144 (-27.0922, 22.2022) -> (-27.0922, 23.3246)
  line L145 (-27.0922, 23.3246) -> (-28.2146, 23.3246)
  line L146 (-28.2146, 23.3246) -> (-28.2146, 22.2022)
  line L147 (-28.2146, 24.4911) -> (-27.0922, 24.4911)
  line L148 (-27.0922, 24.4911) -> (-27.0922, 30.2022)
  line L149 (-27.0922, 30.2022) -> (-28.2146, 30.2022)
  line L150 (-28.2146, 30.2022) -> (-28.2146, 24.4911)
  spline S199 degree 2 poles (-18.564, 26.7414) (-18.564, 26.1362) (-18.8776, 25.8061) knots 0 0 0 1 1 1
  spline S200 degree 2 poles (-18.8776, 25.8061) (-19.1912, 25.4759) (-19.7579, 25.4759) knots 0 0 0 1 1 1
  spline S201 degree 2 poles (-19.7579, 25.4759) (-20.2806, 25.4759) (-20.5667, 25.795) knots 0 0 0 1 1 1
  spline S202 degree 2 poles (-20.5667, 25.795) (-20.8528, 26.1142) (-20.8528, 26.6974) knots 0 0 0 1 1 1
  line L151 (-20.8528, 26.6974) -> (-21.0784, 25.597)
  spline S203 degree 2 poles (-21.0784, 25.597) (-20.8088, 25.0303) (-20.3659, 24.7194) knots 0 0 0 1 1 1
  spline S204 degree 2 poles (-20.3659, 24.7194) (-19.923, 24.4085) (-19.3893, 24.4085) knots 0 0 0 1 1 1
  spline S205 degree 2 poles (-19.3893, 24.4085) (-18.773, 24.4085) (-18.3356, 24.6809) knots 0 0 0 1 1 1
  spline S206 degree 2 poles (-18.3356, 24.6809) (-17.8982, 24.9532) (-17.6699, 25.4759) knots 0 0 0 1 1 1
  spline S207 degree 2 poles (-17.6699, 25.4759) (-17.4415, 25.9986) (-17.4415, 26.7359) knots 0 0 0 1 1 1
  line L152 (-17.4415, 26.7359) -> (-17.4415, 30.2022)
  line L153 (-17.4415, 30.2022) -> (-18.564, 30.2022)
  line L154 (-18.564, 30.2022) -> (-18.564, 26.7414)
  line L155 (-25.3865, 24.4911) -> (-24.2641, 24.4911)
  line L156 (-24.2641, 24.4911) -> (-24.2641, 30.2022)
  line L157 (-24.2641, 30.2022) -> (-25.3865, 30.2022)
  line L158 (-25.3865, 30.2022) -> (-25.3865, 24.4911)
  spline S208 degree 2 poles (-21.9752, 26.7414) (-21.9752, 26.1362) (-22.2724, 25.8061) knots 0 0 0 1 1 1
  spline S209 degree 2 poles (-22.2724, 25.8061) (-22.5695, 25.4759) (-23.1142, 25.4759) knots 0 0 0 1 1 1
  spline S210 degree 2 poles (-23.1142, 25.4759) (-23.6644, 25.4759) (-23.9642, 25.7675) knots 0 0 0 1 1 1
  spline S211 degree 2 poles (-23.9642, 25.7675) (-24.2641, 26.0591) (-24.2641, 26.5873) knots 0 0 0 1 1 1
  line L159 (-24.2641, 26.5873) -> (-24.3796, 25.4869)
  spline S212 degree 2 poles (-24.3796, 25.4869) (-24.1155, 24.9697) (-23.6891, 24.6891) knots 0 0 0 1 1 1
  spline S213 degree 2 poles (-23.6891, 24.6891) (-23.2627, 24.4085) (-22.7455, 24.4085) knots 0 0 0 1 1 1
  spline S214 degree 2 poles (-22.7455, 24.4085) (-22.1458, 24.4085) (-21.7221, 24.6809) knots 0 0 0 1 1 1
  spline S215 degree 2 poles (-21.7221, 24.6809) (-21.2985, 24.9532) (-21.0757, 25.4759) knots 0 0 0 1 1 1
  spline S216 degree 2 poles (-21.0757, 25.4759) (-20.8528, 25.9986) (-20.8528, 26.7359) knots 0 0 0 1 1 1
  line L160 (-20.8528, 26.7359) -> (-20.8528, 30.2022)
  line L161 (-20.8528, 30.2022) -> (-21.9752, 30.2022)
  line L162 (-21.9752, 30.2022) -> (-21.9752, 26.7414)
  spline S217 degree 2 poles (-13.3975, 30.2847) (-14.1898, 30.2847) (-14.751, 29.9876) knots 0 0 0 1 1 1
  spline S218 degree 2 poles (-14.751, 29.9876) (-15.3122, 29.6905) (-15.6066, 29.1155) knots 0 0 0 1 1 1
  spline S219 degree 2 poles (-15.6066, 29.1155) (-15.901, 28.5406) (-15.901, 27.7263) knots 0 0 0 1 1 1
  line L163 (-15.901, 27.7263) -> (-15.901, 27.0825)
  spline S220 degree 2 poles (-15.901, 27.0825) (-15.901, 26.2352) (-15.6176, 25.6355) knots 0 0 0 1 1 1
  spline S221 degree 2 poles (-15.6176, 25.6355) (-15.3342, 25.0358) (-14.795, 24.7221) knots 0 0 0 1 1 1
  spline S222 degree 2 poles (-14.795, 24.7221) (-14.2558, 24.4085) (-13.4966, 24.4085) knots 0 0 0 1 1 1
  spline S223 degree 2 poles (-13.4966, 24.4085) (-12.7813, 24.4085) (-12.2751, 24.7662) knots 0 0 0 1 1 1
  spline S224 degree 2 poles (-12.2751, 24.7662) (-11.7689, 25.1238) (-11.5021, 25.8005) knots 0 0 0 1 1 1
  spline S225 degree 2 poles (-11.5021, 25.8005) (-11.2352, 26.4773) (-11.2352, 27.4237) knots 0 0 0 1 1 1
  line L164 (-11.2352, 27.4237) -> (-11.2352, 27.7978)
  line L165 (-11.2352, 27.7978) -> (-15.0867, 27.7978)
  line L166 (-15.0867, 27.7978) -> (-15.0867, 26.8955)
  line L167 (-15.0867, 26.8955) -> (-12.3026, 26.8955)
  spline S226 degree 2 poles (-12.3026, 26.8955) (-12.3521, 26.1967) (-12.663, 25.8088) knots 0 0 0 1 1 1
  spline S227 degree 2 poles (-12.663, 25.8088) (-12.9739, 25.4209) (-13.4966, 25.4209) knots 0 0 0 1 1 1
  spline S228 degree 2 poles (-13.4966, 25.4209) (-14.1348, 25.4209) (-14.4842, 25.8391) knots 0 0 0 1 1 1
  spline S229 degree 2 poles (-14.4842, 25.8391) (-14.8336, 26.2572) (-14.8336, 27.022) knots 0 0 0 1 1 1
  line L168 (-14.8336, 27.022) -> (-14.8336, 27.7483)
  spline S230 degree 2 poles (-14.8336, 27.7483) (-14.8336, 28.458) (-14.4594, 28.8377) knots 0 0 0 1 1 1
  spline S231 degree 2 poles (-14.4594, 28.8377) (-14.0853, 29.2173) (-13.3975, 29.2173) knots 0 0 0 1 1 1
  spline S232 degree 2 poles (-13.3975, 29.2173) (-13.0564, 29.2173) (-12.7208, 29.0798) knots 0 0 0 1 1 1
  spline S233 degree 2 poles (-12.7208, 29.0798) (-12.3851, 28.9422) (-12.121, 28.6946) knots 0 0 0 1 1 1
  line L169 (-12.121, 28.6946) -> (-11.3838, 29.4319)
  spline S234 degree 2 poles (-11.3838, 29.4319) (-11.8074, 29.8391) (-12.3356, 30.0619) knots 0 0 0 1 1 1
  spline S235 degree 2 poles (-12.3356, 30.0619) (-12.8638, 30.2847) (-13.3975, 30.2847) knots 0 0 0 1 1 1
  line L170 (-9.5791, 22.2077) -> (-8.6988, 22.2077)
  line L171 (-8.6988, 22.2077) -> (-8.6988, 25.0083)
  line L172 (-8.6988, 25.0083) -> (-9.5791, 25.0083)
  line L173 (-9.5791, 25.0083) -> (-9.5791, 22.2077)
  line L174 (-10.63, 21.5805) -> (-7.6479, 21.5805)
  line L175 (-7.6479, 21.5805) -> (-7.6479, 22.4443)
  line L176 (-7.6479, 22.4443) -> (-10.63, 22.4443)
  line L177 (-10.63, 22.4443) -> (-10.63, 21.5805)
  line L178 (-4.5392, 21.5805) -> (-3.7139, 21.5805)
  line L179 (-3.7139, 21.5805) -> (-3.7139, 25.0083)
  line L180 (-3.7139, 25.0083) -> (-4.5392, 25.0083)
  line L181 (-4.5392, 25.0083) -> (-4.5392, 22.9505)
  line L182 (-4.5392, 22.9505) -> (-4.3466, 22.6974)
  line L183 (-4.3466, 22.6974) -> (-5.3535, 24.5846)
  line L184 (-5.3535, 24.5846) -> (-5.5791, 24.5846)
  line L185 (-5.5791, 24.5846) -> (-6.5805, 22.6974)
  line L186 (-6.5805, 22.6974) -> (-6.3934, 22.9505)
  line L187 (-6.3934, 22.9505) -> (-6.3934, 25.0083)
  line L188 (-6.3934, 25.0083) -> (-7.2242, 25.0083)
  line L189 (-7.2242, 25.0083) -> (-7.2242, 21.5805)
  line L190 (-7.2242, 21.5805) -> (-6.3989, 21.5805)
  line L191 (-6.3989, 21.5805) -> (-5.4691, 23.2586)
  line L192 (-5.4691, 23.2586) -> (-4.5392, 21.5805)
  dimension "d1" = 60
  dimension "d2" = 40
  dimension "d10" = 60
  dimension "d11" = 5
  dimension "d13" = 28
  constraint horizontal L0
  constraint vertical L1
  constraint horizontal L2
  constraint vertical L3
  constraint coincident L0.start L3.end
  constraint horizontal L32
  constraint vertical L33
  constraint horizontal L34
  constraint vertical L35
  constraint collinear L3 L35
  measures "d1" distance of L1.end L2.end
  measures "d2" distance of L0.start L2.end
  measures "d10" distance of L32.start L32.end
  measures "d11" distance of L0.start L32.start
  measures "d13" distance of L32.start L34.end
extrude "Extrude1" add sketch "Sketch1" along normal blind 3.5 contours L0 L1 L2 L3 | S0 S1 S2 S3 S4 S5 S6 S7 S8 L5 L6 L7 S17 | L4 S4 S17 | L4 S4 L9 S9 S10 S11 S12 S13 S14 S15 S16 S17 L13 L14 L15 | L9 L12 S13 | L8 L9 L10 L11 L12 S13 | L16 L17 L18 L19 | L20 L21 L22 L23 | L24 L25 L26 L27 S25 L29 L31 S36 | L27 S18 S19 S20 L28 S21 S22 S23 S24 S25 S26 S27 S28 S29 S30 L30 S31 S32 S33 S34 S35 S36 S37 | L27 S25 L29 | L27 S26 S27 S28 S29 S30 L30 S31 S32 S33 S34 S35 | L27 L31 S36 | L32 L33 L34 L35 | S38 S39 S40 L36 S41 S42 S43 S44 S45 S46 L37 S47 S48 S49 S50 S51 S52 L38 S53 S54 S55 S56 S57 S58 L39 S59 S60 S61 | L44 S71 S72 S73 S74 | L42 L43 L44 S74 L45 S75 | S62 S63 S64 L40 S65 S66 S67 S68 S69 S70 L41 L42 S75 S76 S77 S78 L46 S79 S80 | L47 L48 L49 L50 L51 S85 | L48 L51 S85 | L48 S81 S82 S83 S84 S85 S86 S87 S88 L52 | S89 S90 L53 L55 S91 S92 L56 L57 L58 L61 | L53 L55 L59 L61 | L53 L59 L61 L62 | L53 L54 L55 L59 | L55 L59 L60 L61 | L63 L64 L65 L66 | L67 L68 L69 L70 | S93 S94 L71 L72 L73 S95 S96 L74 L76 L77 | L76 L77 L79 L80 | L74 L76 L77 L79 | L74 L75 L76 L79 | L74 L77 L78 L79 | L81 L82 L83 L84 | L85 L86 L87 L88 | L93 S106 S107 S108 S109 | L91 L92 L93 S109 L94 S110 | S97 S98 S99 L89 S100 S101 S102 S103 S104 S105 L90 L91 S110 S111 S112 S113 L95 S114 S115 | L96 L97 L98 L99 S123 L101 L103 S134 | L99 S116 S117 S118 L100 S119 S120 S121 S122 S123 S124 S125 S126 S127 S128 L102 S129 S130 S131 S132 S133 S134 S135 | L99 S123 L101 | L99 S124 S125 S126 S127 S128 L102 S129 S130 S131 S132 S133 | L99 L103 S134 | L104 L113 L114 L116 L117 | L104 L106 L107 L108 L109 L110 L114 L115 L116 L117 L118 | L104 S136 S137 L105 S138 S139 S140 L106 L108 S141 S142 S143 S144 L109 L111 S145 S146 S147 S148 S149 S150 S151 S152 S153 L112 S154 S155 S156 L113 L116 | L104 S136 S137 L105 S138 S139 S140 L106 L116 | L106 L107 L108 L116 | L108 S141 S142 S143 S144 L109 L116 | L109 L110 L111 L115 L116 | S157 S158 S159 S160 L119 S161 S162 S163 S164 S165 L120 L121 L122 L123 L124 L125 L126 S176 | L122 S166 S167 S168 S169 L123 L125 S170 S171 S172 S173 S174 S175 S176 S177 S178 | L122 L123 L124 L125 | L122 L125 S170 S171 S172 S173 S174 S175 | L122 L126 S176 | L127 L128 L129 L130 S186 L132 L134 S197 | L130 S179 S180 S181 L131 S182 S183 S184 S185 S186 S187 S188 S189 S190 S191 L133 S192 S193 S194 S195 S196 S197 S198 | L130 S186 L132 | L130 S187 S188 S189 S190 S191 L133 S192 S193 S194 S195 S196 | L130 L134 S197 | L135 L136 L138 L141 | L135 L136 L138 L139 L140 L141 L142 | L136 L137 L138 L141 | L143 L144 L145 L146 | L147 L148 L149 L150 | S199 S200 S201 S202 S203 S204 S205 S206 S207 L152 L153 L154 S216 | L151 S203 S216 | L151 S203 L156 S208 S209 S210 S211 S212 S213 S214 S215 S216 L160 L161 L162 | L156 L159 S212 | L155 L156 L157 L158 L159 S212 | L167 S226 S227 S228 S229 | L165 L166 L167 S229 L168 S230 | S217 S218 S219 L163 S220 S221 S222 S223 S224 S225 L164 L165 S230 S231 S232 S233 L169 S234 S235 | L170 L171 L173 L176 | L170 L171 L173 L174 L175 L176 L177 | L171 L172 L173 L176 | L181 L182 L183 | L185 L186 L187 | L178 L179 L180 L181 L183 L184 L185 L187 L188 L189 L190 L191 L192 makes body 1 at (-40, 0, 13.3333) makes body 2 at (-20, 0, -14.3333)
extrude "Extrude2" add sketch "Sketch1" against normal blind 1.6 contours S0 S1 S2 S3 S4 S5 S6 S7 S8 L5 L6 L7 S17 | L4 S4 S17 | L4 S4 L9 S9 S10 S11 S12 S13 S14 S15 S16 S17 L13 L14 L15 | L9 L12 S13 | L8 L9 L10 L11 L12 S13 | L16 L17 L18 L19 | L20 L21 L22 L23 | L24 L25 L26 L27 S25 L29 L31 S36 | L27 S18 S19 S20 L28 S21 S22 S23 S24 S25 S26 S27 S28 S29 S30 L30 S31 S32 S33 S34 S35 S36 S37 | L27 S25 L29 | L27 L31 S36 | S38 S39 S40 L36 S41 S42 S43 S44 S45 S46 L37 S47 S48 S49 S50 S51 S52 L38 S53 S54 S55 S56 S57 S58 L39 S59 S60 S61 | L42 L43 L44 S74 L45 S75 | S62 S63 S64 L40 S65 S66 S67 S68 S69 S70 L41 L42 S75 S76 S77 S78 L46 S79 S80 | L47 L48 L49 L50 L51 S85 | L48 L51 S85 | L48 S81 S82 S83 S84 S85 S86 S87 S88 L52 | S89 S90 L53 L55 S91 S92 L56 L57 L58 L61 | L53 L55 L59 L61 | L53 L59 L61 L62 | L53 L54 L55 L59 | L55 L59 L60 L61 | L63 L64 L65 L66 | L67 L68 L69 L70 | S93 S94 L71 L72 L73 S95 S96 L74 L76 L77 | L76 L77 L79 L80 | L74 L76 L77 L79 | L74 L75 L76 L79 | L74 L77 L78 L79 | L81 L82 L83 L84 | L85 L86 L87 L88 | L91 L92 L93 S109 L94 S110 | S97 S98 S99 L89 S100 S101 S102 S103 S104 S105 L90 L91 S110 S111 S112 S113 L95 S114 S115 | L96 L97 L98 L99 S123 L101 L103 S134 | L99 S116 S117 S118 L100 S119 S120 S121 S122 S123 S124 S125 S126 S127 S128 L102 S129 S130 S131 S132 S133 S134 S135 | L99 S123 L101 | L99 L103 S134 | L104 L113 L114 L116 L117 | L104 L106 L107 L108 L109 L110 L114 L115 L116 L117 L118 | L104 S136 S137 L105 S138 S139 S140 L106 L108 S141 S142 S143 S144 L109 L111 S145 S146 S147 S148 S149 S150 S151 S152 S153 L112 S154 S155 S156 L113 L116 | L106 L107 L108 L116 | L109 L110 L111 L115 L116 | S157 S158 S159 S160 L119 S161 S162 S163 S164 S165 L120 L121 L122 L123 L124 L125 L126 S176 | L122 S166 S167 S168 S169 L123 L125 S170 S171 S172 S173 S174 S175 S176 S177 S178 | L122 L123 L124 L125 | L122 L126 S176 | L127 L128 L129 L130 S186 L132 L134 S197 | L130 S179 S180 S181 L131 S182 S183 S184 S185 S186 S187 S188 S189 S190 S191 L133 S192 S193 S194 S195 S196 S197 S198 | L130 S186 L132 | L130 L134 S197 | L135 L136 L138 L141 | L135 L136 L138 L139 L140 L141 L142 | L136 L137 L138 L141 | L143 L144 L145 L146 | L147 L148 L149 L150 | S199 S200 S201 S202 S203 S204 S205 S206 S207 L152 L153 L154 S216 | L151 S203 S216 | L151 S203 L156 S208 S209 S210 S211 S212 S213 S214 S215 S216 L160 L161 L162 | L156 L159 S212 | L155 L156 L157 L158 L159 S212 | L165 L166 L167 S229 L168 S230 | S217 S218 S219 L163 S220 S221 S222 S223 S224 S225 L164 L165 S230 S231 S232 S233 L169 S234 S235 | L170 L171 L173 L176 | L170 L171 L173 L174 L175 L176 L177 | L171 L172 L173 L176 | L181 L182 L183 | L185 L186 L187 | L178 L179 L180 L181 L183 L184 L185 L187 L188 L189 L190 L191 L192 bodies 1 2
fillet "Fillet1" radius 10 4 edges at (-60, 1.75, 40) (-60, 1.75, 0) (0, 1.75, 0) (0, 1.75, 40) on bodies 1
fillet "Fillet2" radius 5 4 edges at (-60, 1.75, -5) (-60, 1.75, -33) (0, 1.75, -33) (0, 1.75, -5) on bodies 2
equation "d10 = d1"
